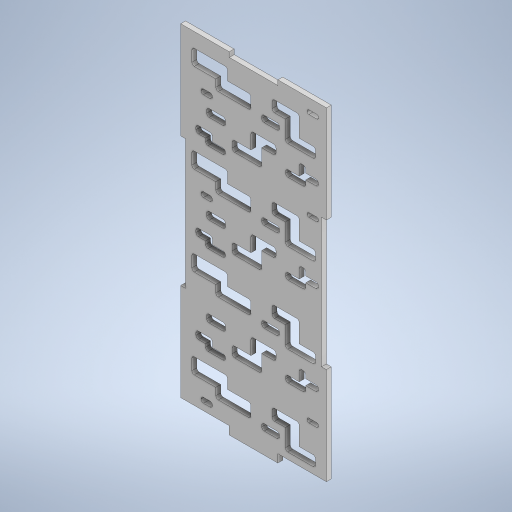
# Autodesk Inventor part: Pièce Ve1
Saved by Autodesk Inventor 2023 (Build 270158000, 158)
## iProperties
Created: 2025-01-14
Part Number: Pièce Ve1
Material: Générique
Document SubType Name: Modeling
Designer: kfadieieva
Density: 1 g/cm^3
Appearance: Par défaut
Author: kfadieieva
Autodesk Inventor part; units mm, degrees
ref_plane "YZ Plane" through (0, 0, 0) normal (1, 0, 0) x (0, 1, 0)
ref_plane "XZ Plane" through (0, 0, 0) normal (0, 1, 0) x (-1, 0, 0)
ref_plane "XY Plane" through (0, 0, 0) normal (0, 0, 1) x (1, 0, 0)
sketch "Esquisse1" plane through (0, 0, 0) normal (0, 0, 1) x (1, 0, 0)
  line L0 (30, 200) -> (30, 197)
  line L1 (30, 197) -> (60, 197)
  line L2 (60, 197) -> (60, 200)
  line L3 (90, 140) -> (87, 140)
  line L4 (87, 140) -> (87, 60)
  line L5 (87, 60) -> (90, 60)
  line L6 (0, 140) -> (3, 140)
  line L7 (3, 140) -> (3, 60)
  line L8 (3, 60) -> (0, 60)
  line L9 (0, 200) -> (0, 140)
  line L10 (0, 60) -> (0, 0)
  line L11 (90, 0) -> (90, 60)
  line L12 (90, 140) -> (90, 200)
  line L13 (90, 200) -> (60, 200)
  line L14 (30, 200) -> (0, 200)
  line L15 (60, 0) -> (60, -5)
  line L16 (60, -5) -> (30, -5)
  line L17 (30, -5) -> (30, 0)
  line L18 (0, 0) -> (30, 0)
  line L19 (60, 0) -> (90, 0)
  dimension "d0" = 90
  dimension "d1" = 200
  dimension "d6" = 200
  dimension "d11" = 3
  dimension "d12" = 3
  dimension "d29" = 30
  dimension "d30" = 3
  dimension "d32" = 30
  dimension "d33" = 30
  dimension "d34" = 90
  dimension "d35" = 90
  dimension "d36" = 90
  dimension "d37" = 90
  dimension "d38" = 90
  dimension "d39" = 90
  dimension "d40" = 90
  dimension "d41" = 5
  dimension "d42" = 90
  dimension "d43" = 90
  dimension "d44" = 90
  dimension "d45" = 90
  dimension "d46" = 90
  constraints: 40 end point, 10 perpendicular, 8 parallel, 3 horizontal, 2 point on line, 1 vertical
  measures "d0" distance of L12.end L9.start
  measures "d1" distance of L11.start L12.end
  measures "d6" distance of L9.start L10.end
  measures "d11" distance of L3.start L3.end
  measures "d12" distance of L1.end L2.end
  measures "d29" distance from line of L9 L0.start
  measures "d30" distance of L6.start L6.end
  measures "d32" distance from line of L16.end L10
  measures "d33" distance from line of L11 L15.end
  measures "d34" angle of L12 L13
  measures "d35" angle of L9 L14
  measures "d36" angle of L0 L14
  measures "d37" angle of L13 L2
  measures "d38" angle of L6 L9
  measures "d39" angle of L10 L8
  measures "d40" angle of L18 L10
  measures "d41" distance of L16.end L17.end
  measures "d42" angle of L19 L15
  measures "d43" angle of L17 L18
  measures "d44" angle of L11 L19
  measures "d45" angle of L11 L5
  measures "d46" angle of L12 L3
extrude "Extrusion1" add sketch "Esquisse1" along normal blind 3
sketch "Esquisse2" plane through (0, 0, 3) normal (0, 0, 1) x (1, 0, 0)
  line L0 (8.393, 191.0718) -> (27.4432, 191.0718)
  line L1 (28.9432, 189.5718) -> (28.9432, 183.8393)
  line L2 (21.7107, 181.3697) -> (8.393, 181.3697)
  line L3 (6.893, 182.8697) -> (6.893, 189.5718)
  line L4 (23.2107, 175.372) -> (41.9082, 175.372)
  line L5 (43.4082, 176.872) -> (43.4082, 182.3393)
  line L6 (41.9082, 183.8393) -> (28.9432, 183.8393)
  line L7 (21.7107, 181.3697) -> (21.7107, 176.872)
  line L8 (57.9619, 188.2494) -> (71.7201, 188.2494)
  line L9 (73.2201, 186.7494) -> (73.2201, 181.3697)
  line L10 (73.2201, 181.3697) -> (57.9619, 181.3697)
  line L11 (56.4619, 182.8697) -> (56.4619, 186.7494)
  line L12 (64.664, 186.2208) -> (73.2201, 186.2208)
  line L13 (73.2201, 186.2208) -> (73.2201, 169.0216)
  line L14 (73.2201, 169.0216) -> (66.164, 169.0216)
  line L15 (64.664, 170.5216) -> (64.664, 186.2208)
  line L16 (69.6921, 169.0216) -> (81.775, 169.0216)
  line L17 (83.275, 170.5216) -> (83.275, 173.872)
  line L18 (81.775, 175.372) -> (69.6921, 175.372)
  line L19 (69.6921, 175.372) -> (69.6921, 169.0216)
  line L20 (14.0378, 172.1968) -> (18.0939, 172.1968)
  line L21 (19.5939, 170.6968) -> (19.5939, 170.5216)
  line L22 (18.0939, 169.0216) -> (14.0378, 169.0216)
  line L23 (12.5378, 170.5216) -> (12.5378, 170.6968)
  line L24 (44.9082, 164.3786) -> (57.362, 164.3786)
  line L25 (58.862, 162.8786) -> (58.862, 160.2175)
  line L26 (57.362, 158.7175) -> (50.0557, 158.7175)
  line L27 (43.4082, 158.7175) -> (43.4082, 162.8786)
  line L28 (50.0557, 158.7175) -> (50.0557, 149.3984)
  line L29 (48.5557, 147.8984) -> (43.4082, 147.8984)
  line L30 (43.4082, 154.1885) -> (43.4082, 162.24)
  line L31 (45.401, 147.8984) -> (33.3142, 147.8984)
  line L32 (31.8142, 149.3984) -> (31.8142, 152.6885)
  line L33 (33.3142, 154.1885) -> (43.4082, 154.1885)
  line L34 (66.341, 155.0692) -> (73.2201, 155.0692)
  line L35 (77.2292, 155.0692) -> (77.2292, 152.5435)
  line L36 (75.7292, 151.0435) -> (66.341, 151.0435)
  line L37 (64.841, 152.5435) -> (64.841, 153.5692)
  line L38 (73.2201, 155.0692) -> (73.2201, 160.798)
  line L39 (74.7201, 162.298) -> (75.7292, 162.298)
  line L40 (77.2292, 158.7175) -> (83.529, 158.7175)
  line L41 (85.029, 157.2175) -> (85.029, 156.5692)
  line L42 (83.529, 155.0692) -> (77.2292, 155.0692)
  line L43 (26.1359, 163.4585) -> (17.5659, 163.4585)
  line L44 (16.0659, 161.9585) -> (16.0659, 160.2175)
  line L45 (17.5659, 158.7175) -> (26.1359, 158.7175)
  line L46 (27.6359, 160.2175) -> (27.6359, 161.9585)
  line L47 (10.9302, 151.0435) -> (18.0939, 151.0435)
  line L48 (19.5939, 149.5435) -> (19.5939, 146.5532)
  line L49 (15.3904, 146.5532) -> (10.9302, 146.5532)
  line L50 (9.4302, 148.0532) -> (9.4302, 149.5435)
  line L51 (19.5939, 146.5532) -> (26.1359, 146.5532)
  line L52 (27.6359, 145.0532) -> (27.6359, 144.6939)
  line L53 (26.1359, 143.1939) -> (16.8904, 143.1939)
  line L54 (15.3904, 144.6939) -> (15.3904, 146.5532)
  line L55 (79.141, 193.6205) -> (84.029, 193.6205)
  line L56 (85.029, 192.6205) -> (85.029, 192.0718)
  line L57 (84.029, 191.0718) -> (79.141, 191.0718)
  line L58 (78.141, 192.0718) -> (78.141, 192.6205)
  arc A0 (8.393, 191.0718) -> (6.893, 189.5718) centre (8.393, 189.5718) ccw
  arc A1 (6.893, 182.8697) -> (8.393, 181.3697) centre (8.393, 182.8697) ccw
  arc A2 (14.0378, 172.1968) -> (12.5378, 170.6968) centre (14.0378, 170.6968) ccw
  arc A3 (12.5378, 170.5216) -> (14.0378, 169.0216) centre (14.0378, 170.5216) ccw
  arc A4 (19.5939, 170.6968) -> (18.0939, 172.1968) centre (18.0939, 170.6968) ccw
  arc A5 (18.0939, 169.0216) -> (19.5939, 170.5216) centre (18.0939, 170.5216) ccw
  arc A6 (27.6359, 161.9585) -> (26.1359, 163.4585) centre (26.1359, 161.9585) ccw
  arc A7 (26.1359, 158.7175) -> (27.6359, 160.2175) centre (26.1359, 160.2175) ccw
  arc A8 (16.0659, 160.2175) -> (17.5659, 158.7175) centre (17.5659, 160.2175) ccw
  arc A9 (17.5659, 163.4585) -> (16.0659, 161.9585) centre (17.5659, 161.9585) ccw
  arc A10 (10.9302, 151.0435) -> (9.4302, 149.5435) centre (10.9302, 149.5435) ccw
  arc A11 (9.4302, 148.0532) -> (10.9302, 146.5532) centre (10.9302, 148.0532) ccw
  arc A12 (19.5939, 149.5435) -> (18.0939, 151.0435) centre (18.0939, 149.5435) ccw
  arc A13 (15.3904, 144.6939) -> (16.8904, 143.1939) centre (16.8904, 144.6939) ccw
  arc A14 (26.1359, 143.1939) -> (27.6359, 144.6939) centre (26.1359, 144.6939) ccw
  arc A15 (27.6359, 145.0532) -> (26.1359, 146.5532) centre (26.1359, 145.0532) ccw
  arc A16 (33.3142, 154.1885) -> (31.8142, 152.6885) centre (33.3142, 152.6885) ccw
  arc A17 (31.8142, 149.3984) -> (33.3142, 147.8984) centre (33.3142, 149.3984) ccw
  arc A18 (44.9082, 164.3786) -> (43.4082, 162.8786) centre (44.9082, 162.8786) ccw
  arc A19 (57.362, 158.7175) -> (58.862, 160.2175) centre (57.362, 160.2175) ccw
  arc A20 (58.862, 162.8786) -> (57.362, 164.3786) centre (57.362, 162.8786) ccw
  arc A21 (48.5557, 147.8984) -> (50.0557, 149.3984) centre (48.5557, 149.3984) ccw
  arc A22 (66.341, 155.0692) -> (64.841, 153.5692) centre (66.341, 153.5692) ccw
  arc A23 (64.841, 152.5435) -> (66.341, 151.0435) centre (66.341, 152.5435) ccw
  arc A24 (75.7292, 151.0435) -> (77.2292, 152.5435) centre (75.7292, 152.5435) ccw
  arc A25 (83.529, 155.0692) -> (85.029, 156.5692) centre (83.529, 156.5692) ccw
  arc A26 (85.029, 157.2175) -> (83.529, 158.7175) centre (83.529, 157.2175) ccw
  arc A27 (77.2292, 160.798) -> (75.7292, 162.298) centre (75.7292, 160.798) ccw
  arc A28 (74.7201, 162.298) -> (73.2201, 160.798) centre (74.7201, 160.798) ccw
  arc A29 (28.9432, 189.5718) -> (27.4432, 191.0718) centre (27.4432, 189.5718) ccw
  arc A30 (21.7107, 176.872) -> (23.2107, 175.372) centre (23.2107, 176.872) ccw
  arc A31 (41.9082, 175.372) -> (43.4082, 176.872) centre (41.9082, 176.872) ccw
  arc A32 (43.4082, 182.3393) -> (41.9082, 183.8393) centre (41.9082, 182.3393) ccw
  arc A33 (57.9619, 188.2494) -> (56.4619, 186.7494) centre (57.9619, 186.7494) ccw
  arc A34 (56.4619, 182.8697) -> (57.9619, 181.3697) centre (57.9619, 182.8697) ccw
  arc A35 (73.2201, 186.7494) -> (71.7201, 188.2494) centre (71.7201, 186.7494) ccw
  arc A36 (64.664, 170.5216) -> (66.164, 169.0216) centre (66.164, 170.5216) ccw
  arc A37 (81.775, 169.0216) -> (83.275, 170.5216) centre (81.775, 170.5216) ccw
  arc A38 (83.275, 173.872) -> (81.775, 175.372) centre (81.775, 173.872) ccw
  line L59 (51.5557, 176.872) -> (59.471, 176.872)
  line L60 (60.971, 175.372) -> (60.971, 174.415)
  line L61 (59.471, 172.915) -> (51.5557, 172.915)
  line L62 (50.0557, 174.415) -> (50.0557, 175.372)
  arc A39 (51.5557, 176.872) -> (50.0557, 175.372) centre (51.5557, 175.372) ccw
  arc A40 (50.0557, 174.415) -> (51.5557, 172.915) centre (51.5557, 174.415) ccw
  arc A41 (59.471, 172.915) -> (60.971, 174.415) centre (59.471, 174.415) ccw
  arc A42 (60.971, 175.372) -> (59.471, 176.872) centre (59.471, 175.372) ccw
  arc A43 (79.141, 193.6205) -> (78.141, 192.6205) centre (79.141, 192.6205) ccw
  arc A44 (78.141, 192.0718) -> (79.141, 191.0718) centre (79.141, 192.0718) ccw
  arc A45 (85.029, 192.6205) -> (84.029, 193.6205) centre (84.029, 192.6205) ccw
  arc A46 (84.029, 191.0718) -> (85.029, 192.0718) centre (84.029, 192.0718) ccw
  line L63 (43.4082, 162.24) -> (43.5509, 162.24)
  line L64 (77.2292, 160.798) -> (77.2292, 158.7175)
  line L65 (77.2292, 155.0692) -> (77.2292, 153.8063)
  arc A47 (6.893, 127.8697) -> (8.393, 126.3697) centre (8.393, 127.8697) ccw
  line L66 (6.893, 127.8697) -> (6.893, 134.5718)
  arc A48 (8.393, 136.0718) -> (6.893, 134.5718) centre (8.393, 134.5718) ccw
  line L67 (12.5378, 115.5216) -> (12.5378, 115.6968)
  line L68 (66.341, 100.0692) -> (73.2201, 100.0692)
  line L69 (77.2292, 100.0692) -> (77.2292, 97.5435)
  line L70 (75.7292, 96.0435) -> (66.341, 96.0435)
  line L71 (77.2292, 100.0692) -> (77.2292, 98.8063)
  arc A49 (75.7292, 96.0435) -> (77.2292, 97.5435) centre (75.7292, 97.5435) ccw
  line L72 (83.529, 100.0692) -> (77.2292, 100.0692)
  line L73 (77.2292, 105.798) -> (77.2292, 103.7175)
  line L74 (73.2201, 100.0692) -> (73.2201, 105.798)
  line L75 (74.7201, 107.298) -> (75.7292, 107.298)
  arc A50 (74.7201, 107.298) -> (73.2201, 105.798) centre (74.7201, 105.798) ccw
  arc A51 (77.2292, 105.798) -> (75.7292, 107.298) centre (75.7292, 105.798) ccw
  line L76 (77.2292, 103.7175) -> (83.529, 103.7175)
  line L77 (10.9302, 96.0435) -> (18.0939, 96.0435)
  line L78 (15.3904, 91.5532) -> (10.9302, 91.5532)
  line L79 (9.4302, 93.0532) -> (9.4302, 94.5435)
  arc A52 (10.9302, 96.0435) -> (9.4302, 94.5435) centre (10.9302, 94.5435) ccw
  arc A53 (9.4302, 93.0532) -> (10.9302, 91.5532) centre (10.9302, 93.0532) ccw
  line L80 (15.3904, 89.6939) -> (15.3904, 91.5532)
  line L81 (57.9619, 133.2494) -> (71.7201, 133.2494)
  line L82 (73.2201, 131.7494) -> (73.2201, 126.3697)
  line L83 (73.2201, 126.3697) -> (57.9619, 126.3697)
  line L84 (64.664, 131.2208) -> (73.2201, 131.2208)
  line L85 (73.2201, 131.2208) -> (73.2201, 114.0216)
  line L86 (73.2201, 114.0216) -> (66.164, 114.0216)
  line L87 (64.664, 115.5216) -> (64.664, 131.2208)
  line L88 (69.6921, 114.0216) -> (81.775, 114.0216)
  line L89 (83.275, 115.5216) -> (83.275, 118.872)
  line L90 (81.775, 120.372) -> (69.6921, 120.372)
  line L91 (69.6921, 120.372) -> (69.6921, 114.0216)
  arc A54 (73.2201, 131.7494) -> (71.7201, 133.2494) centre (71.7201, 131.7494) ccw
  arc A55 (83.275, 118.872) -> (81.775, 120.372) centre (81.775, 118.872) ccw
  arc A56 (81.775, 114.0216) -> (83.275, 115.5216) centre (81.775, 115.5216) ccw
  arc A57 (14.0378, 117.1968) -> (12.5378, 115.6968) centre (14.0378, 115.6968) ccw
  arc A58 (12.5378, 115.5216) -> (14.0378, 114.0216) centre (14.0378, 115.5216) ccw
  line L92 (8.393, 136.0718) -> (27.4432, 136.0718)
  line L93 (21.7107, 126.3697) -> (8.393, 126.3697)
  line L94 (14.0378, 117.1968) -> (18.0939, 117.1968)
  arc A59 (19.5939, 115.6968) -> (18.0939, 117.1968) centre (18.0939, 115.6968) ccw
  line L95 (19.5939, 115.6968) -> (19.5939, 115.5216)
  line L96 (18.0939, 114.0216) -> (14.0378, 114.0216)
  arc A60 (18.0939, 114.0216) -> (19.5939, 115.5216) centre (18.0939, 115.5216) ccw
  line L97 (26.1359, 108.4585) -> (17.5659, 108.4585)
  line L98 (16.0659, 106.9585) -> (16.0659, 105.2175)
  line L99 (17.5659, 103.7175) -> (26.1359, 103.7175)
  line L100 (27.6359, 105.2175) -> (27.6359, 106.9585)
  arc A61 (17.5659, 108.4585) -> (16.0659, 106.9585) centre (17.5659, 106.9585) ccw
  arc A62 (16.0659, 105.2175) -> (17.5659, 103.7175) centre (17.5659, 105.2175) ccw
  arc A63 (27.6359, 106.9585) -> (26.1359, 108.4585) centre (26.1359, 106.9585) ccw
  arc A64 (26.1359, 103.7175) -> (27.6359, 105.2175) centre (26.1359, 105.2175) ccw
  line L101 (44.9082, 109.3786) -> (57.362, 109.3786)
  line L102 (58.862, 107.8786) -> (58.862, 105.2175)
  line L103 (57.362, 103.7175) -> (50.0557, 103.7175)
  line L104 (64.841, 97.5435) -> (64.841, 98.5692)
  arc A65 (57.362, 103.7175) -> (58.862, 105.2175) centre (57.362, 105.2175) ccw
  arc A66 (58.862, 107.8786) -> (57.362, 109.3786) centre (57.362, 107.8786) ccw
  arc A67 (66.341, 100.0692) -> (64.841, 98.5692) centre (66.341, 98.5692) ccw
  arc A68 (64.664, 115.5216) -> (66.164, 114.0216) centre (66.164, 115.5216) ccw
  arc A69 (64.841, 97.5435) -> (66.341, 96.0435) centre (66.341, 97.5435) ccw
  line L105 (28.9432, 134.5718) -> (28.9432, 128.8393)
  line L106 (23.2107, 120.372) -> (41.9082, 120.372)
  line L107 (43.4082, 121.872) -> (43.4082, 127.3393)
  line L108 (41.9082, 128.8393) -> (28.9432, 128.8393)
  line L109 (21.7107, 126.3697) -> (21.7107, 121.872)
  arc A70 (28.9432, 134.5718) -> (27.4432, 136.0718) centre (27.4432, 134.5718) ccw
  arc A71 (21.7107, 121.872) -> (23.2107, 120.372) centre (23.2107, 121.872) ccw
  arc A72 (41.9082, 120.372) -> (43.4082, 121.872) centre (41.9082, 121.872) ccw
  arc A73 (43.4082, 127.3393) -> (41.9082, 128.8393) centre (41.9082, 127.3393) ccw
  line L110 (56.4619, 127.8697) -> (56.4619, 131.7494)
  line L111 (50.0557, 119.415) -> (50.0557, 120.372)
  arc A74 (51.5557, 121.872) -> (50.0557, 120.372) centre (51.5557, 120.372) ccw
  arc A75 (50.0557, 119.415) -> (51.5557, 117.915) centre (51.5557, 119.415) ccw
  arc A76 (57.9619, 133.2494) -> (56.4619, 131.7494) centre (57.9619, 131.7494) ccw
  arc A77 (56.4619, 127.8697) -> (57.9619, 126.3697) centre (57.9619, 127.8697) ccw
  line L112 (51.5557, 121.872) -> (59.471, 121.872)
  line L113 (59.471, 117.915) -> (51.5557, 117.915)
  line L114 (60.971, 120.372) -> (60.971, 119.415)
  arc A78 (59.471, 117.915) -> (60.971, 119.415) centre (59.471, 119.415) ccw
  arc A79 (60.971, 120.372) -> (59.471, 121.872) centre (59.471, 120.372) ccw
  line L115 (43.4082, 103.7175) -> (43.4082, 107.8786)
  line L116 (50.0557, 103.7175) -> (50.0557, 94.3984)
  line L117 (48.5557, 92.8984) -> (43.4082, 92.8984)
  line L118 (43.4082, 99.1885) -> (43.4082, 107.24)
  line L119 (45.401, 92.8984) -> (33.3142, 92.8984)
  line L120 (31.8142, 94.3984) -> (31.8142, 97.6885)
  line L121 (33.3142, 99.1885) -> (43.4082, 99.1885)
  arc A80 (33.3142, 99.1885) -> (31.8142, 97.6885) centre (33.3142, 97.6885) ccw
  arc A81 (31.8142, 94.3984) -> (33.3142, 92.8984) centre (33.3142, 94.3984) ccw
  arc A82 (44.9082, 109.3786) -> (43.4082, 107.8786) centre (44.9082, 107.8786) ccw
  arc A83 (48.5557, 92.8984) -> (50.0557, 94.3984) centre (48.5557, 94.3984) ccw
  line L122 (43.4082, 107.24) -> (43.5509, 107.24)
  line L123 (19.5939, 94.5435) -> (19.5939, 91.5532)
  arc A84 (15.3904, 89.6939) -> (16.8904, 88.1939) centre (16.8904, 89.6939) ccw
  arc A85 (19.5939, 94.5435) -> (18.0939, 96.0435) centre (18.0939, 94.5435) ccw
  line L124 (26.1359, 88.1939) -> (16.8904, 88.1939)
  line L125 (19.5939, 91.5532) -> (26.1359, 91.5532)
  arc A86 (27.6359, 90.0532) -> (26.1359, 91.5532) centre (26.1359, 90.0532) ccw
  line L126 (27.6359, 90.0532) -> (27.6359, 89.6939)
  arc A87 (26.1359, 88.1939) -> (27.6359, 89.6939) centre (26.1359, 89.6939) ccw
  arc A88 (85.029, 102.2175) -> (83.529, 103.7175) centre (83.529, 102.2175) ccw
  line L127 (85.029, 102.2175) -> (85.029, 101.5692)
  arc A89 (83.529, 100.0692) -> (85.029, 101.5692) centre (83.529, 101.5692) ccw
  line L128 (84.029, 136.0718) -> (79.141, 136.0718)
  arc A90 (78.141, 137.0718) -> (79.141, 136.0718) centre (79.141, 137.0718) ccw
  line L129 (78.141, 137.0718) -> (78.141, 137.6205)
  arc A91 (84.029, 136.0718) -> (85.029, 137.0718) centre (84.029, 137.0718) ccw
  line L130 (85.029, 137.6205) -> (85.029, 137.0718)
  line L131 (79.141, 138.6205) -> (84.029, 138.6205)
  arc A92 (85.029, 137.6205) -> (84.029, 138.6205) centre (84.029, 137.6205) ccw
  arc A93 (79.141, 138.6205) -> (78.141, 137.6205) centre (79.141, 137.6205) ccw
  arc A94 (6.893, 72.8697) -> (8.393, 71.3697) centre (8.393, 72.8697) ccw
  line L132 (6.893, 72.8697) -> (6.893, 79.5718)
  arc A95 (8.393, 81.0718) -> (6.893, 79.5718) centre (8.393, 79.5718) ccw
  line L133 (12.5378, 60.5216) -> (12.5378, 60.6968)
  line L134 (66.341, 45.0692) -> (73.2201, 45.0692)
  line L135 (77.2292, 45.0692) -> (77.2292, 42.5435)
  line L136 (75.7292, 41.0435) -> (66.341, 41.0435)
  line L137 (77.2292, 45.0692) -> (77.2292, 43.8063)
  arc A96 (75.7292, 41.0435) -> (77.2292, 42.5435) centre (75.7292, 42.5435) ccw
  line L138 (83.529, 45.0692) -> (77.2292, 45.0692)
  line L139 (77.2292, 50.798) -> (77.2292, 48.7175)
  line L140 (73.2201, 45.0692) -> (73.2201, 50.798)
  line L141 (74.7201, 52.298) -> (75.7292, 52.298)
  arc A97 (74.7201, 52.298) -> (73.2201, 50.798) centre (74.7201, 50.798) ccw
  arc A98 (77.2292, 50.798) -> (75.7292, 52.298) centre (75.7292, 50.798) ccw
  line L142 (77.2292, 48.7175) -> (83.529, 48.7175)
  line L143 (10.9302, 41.0435) -> (18.0939, 41.0435)
  line L144 (15.3904, 36.5532) -> (10.9302, 36.5532)
  line L145 (9.4302, 38.0532) -> (9.4302, 39.5435)
  arc A99 (10.9302, 41.0435) -> (9.4302, 39.5435) centre (10.9302, 39.5435) ccw
  arc A100 (9.4302, 38.0532) -> (10.9302, 36.5532) centre (10.9302, 38.0532) ccw
  line L146 (15.3904, 34.6939) -> (15.3904, 36.5532)
  line L147 (57.9619, 78.2494) -> (71.7201, 78.2494)
  line L148 (73.2201, 76.7494) -> (73.2201, 71.3697)
  line L149 (73.2201, 71.3697) -> (57.9619, 71.3697)
  line L150 (64.664, 76.2208) -> (73.2201, 76.2208)
  line L151 (73.2201, 76.2208) -> (73.2201, 59.0216)
  line L152 (73.2201, 59.0216) -> (66.164, 59.0216)
  line L153 (64.664, 60.5216) -> (64.664, 76.2208)
  line L154 (69.6921, 59.0216) -> (81.775, 59.0216)
  line L155 (83.275, 60.5216) -> (83.275, 63.872)
  line L156 (81.775, 65.372) -> (69.6921, 65.372)
  line L157 (69.6921, 65.372) -> (69.6921, 59.0216)
  arc A101 (73.2201, 76.7494) -> (71.7201, 78.2494) centre (71.7201, 76.7494) ccw
  arc A102 (83.275, 63.872) -> (81.775, 65.372) centre (81.775, 63.872) ccw
  arc A103 (81.775, 59.0216) -> (83.275, 60.5216) centre (81.775, 60.5216) ccw
  arc A104 (14.0378, 62.1968) -> (12.5378, 60.6968) centre (14.0378, 60.6968) ccw
  arc A105 (12.5378, 60.5216) -> (14.0378, 59.0216) centre (14.0378, 60.5216) ccw
  line L158 (8.393, 81.0718) -> (27.4432, 81.0718)
  line L159 (21.7107, 71.3697) -> (8.393, 71.3697)
  line L160 (14.0378, 62.1968) -> (18.0939, 62.1968)
  arc A106 (19.5939, 60.6968) -> (18.0939, 62.1968) centre (18.0939, 60.6968) ccw
  line L161 (19.5939, 60.6968) -> (19.5939, 60.5216)
  line L162 (18.0939, 59.0216) -> (14.0378, 59.0216)
  arc A107 (18.0939, 59.0216) -> (19.5939, 60.5216) centre (18.0939, 60.5216) ccw
  line L163 (26.1359, 53.4585) -> (17.5659, 53.4585)
  line L164 (16.0659, 51.9585) -> (16.0659, 50.2175)
  line L165 (17.5659, 48.7175) -> (26.1359, 48.7175)
  line L166 (27.6359, 50.2175) -> (27.6359, 51.9585)
  arc A108 (17.5659, 53.4585) -> (16.0659, 51.9585) centre (17.5659, 51.9585) ccw
  arc A109 (16.0659, 50.2175) -> (17.5659, 48.7175) centre (17.5659, 50.2175) ccw
  arc A110 (27.6359, 51.9585) -> (26.1359, 53.4585) centre (26.1359, 51.9585) ccw
  arc A111 (26.1359, 48.7175) -> (27.6359, 50.2175) centre (26.1359, 50.2175) ccw
  line L167 (44.9082, 54.3786) -> (57.362, 54.3786)
  line L168 (58.862, 52.8786) -> (58.862, 50.2175)
  line L169 (57.362, 48.7175) -> (50.0557, 48.7175)
  line L170 (64.841, 42.5435) -> (64.841, 43.5692)
  arc A112 (57.362, 48.7175) -> (58.862, 50.2175) centre (57.362, 50.2175) ccw
  arc A113 (58.862, 52.8786) -> (57.362, 54.3786) centre (57.362, 52.8786) ccw
  arc A114 (66.341, 45.0692) -> (64.841, 43.5692) centre (66.341, 43.5692) ccw
  arc A115 (64.664, 60.5216) -> (66.164, 59.0216) centre (66.164, 60.5216) ccw
  arc A116 (64.841, 42.5435) -> (66.341, 41.0435) centre (66.341, 42.5435) ccw
  line L171 (28.9432, 79.5718) -> (28.9432, 73.8393)
  line L172 (23.2107, 65.372) -> (41.9082, 65.372)
  line L173 (43.4082, 66.872) -> (43.4082, 72.3393)
  line L174 (41.9082, 73.8393) -> (28.9432, 73.8393)
  line L175 (21.7107, 71.3697) -> (21.7107, 66.872)
  arc A117 (28.9432, 79.5718) -> (27.4432, 81.0718) centre (27.4432, 79.5718) ccw
  arc A118 (21.7107, 66.872) -> (23.2107, 65.372) centre (23.2107, 66.872) ccw
  arc A119 (41.9082, 65.372) -> (43.4082, 66.872) centre (41.9082, 66.872) ccw
  arc A120 (43.4082, 72.3393) -> (41.9082, 73.8393) centre (41.9082, 72.3393) ccw
  line L176 (56.4619, 72.8697) -> (56.4619, 76.7494)
  line L177 (50.0557, 64.415) -> (50.0557, 65.372)
  arc A121 (51.5557, 66.872) -> (50.0557, 65.372) centre (51.5557, 65.372) ccw
  arc A122 (50.0557, 64.415) -> (51.5557, 62.915) centre (51.5557, 64.415) ccw
  arc A123 (57.9619, 78.2494) -> (56.4619, 76.7494) centre (57.9619, 76.7494) ccw
  arc A124 (56.4619, 72.8697) -> (57.9619, 71.3697) centre (57.9619, 72.8697) ccw
  line L178 (51.5557, 66.872) -> (59.471, 66.872)
  line L179 (59.471, 62.915) -> (51.5557, 62.915)
  line L180 (60.971, 65.372) -> (60.971, 64.415)
  arc A125 (59.471, 62.915) -> (60.971, 64.415) centre (59.471, 64.415) ccw
  arc A126 (60.971, 65.372) -> (59.471, 66.872) centre (59.471, 65.372) ccw
  line L181 (43.4082, 48.7175) -> (43.4082, 52.8786)
  line L182 (50.0557, 48.7175) -> (50.0557, 39.3984)
  line L183 (48.5557, 37.8984) -> (43.4082, 37.8984)
  line L184 (43.4082, 44.1885) -> (43.4082, 52.24)
  line L185 (45.401, 37.8984) -> (33.3142, 37.8984)
  line L186 (31.8142, 39.3984) -> (31.8142, 42.6885)
  line L187 (33.3142, 44.1885) -> (43.4082, 44.1885)
  arc A127 (33.3142, 44.1885) -> (31.8142, 42.6885) centre (33.3142, 42.6885) ccw
  arc A128 (31.8142, 39.3984) -> (33.3142, 37.8984) centre (33.3142, 39.3984) ccw
  arc A129 (44.9082, 54.3786) -> (43.4082, 52.8786) centre (44.9082, 52.8786) ccw
  arc A130 (48.5557, 37.8984) -> (50.0557, 39.3984) centre (48.5557, 39.3984) ccw
  line L188 (43.4082, 52.24) -> (43.5509, 52.24)
  line L189 (19.5939, 39.5435) -> (19.5939, 36.5532)
  arc A131 (15.3904, 34.6939) -> (16.8904, 33.1939) centre (16.8904, 34.6939) ccw
  arc A132 (19.5939, 39.5435) -> (18.0939, 41.0435) centre (18.0939, 39.5435) ccw
  line L190 (26.1359, 33.1939) -> (16.8904, 33.1939)
  line L191 (19.5939, 36.5532) -> (26.1359, 36.5532)
  arc A133 (27.6359, 35.0532) -> (26.1359, 36.5532) centre (26.1359, 35.0532) ccw
  line L192 (27.6359, 35.0532) -> (27.6359, 34.6939)
  arc A134 (26.1359, 33.1939) -> (27.6359, 34.6939) centre (26.1359, 34.6939) ccw
  arc A135 (85.029, 47.2175) -> (83.529, 48.7175) centre (83.529, 47.2175) ccw
  line L193 (85.029, 47.2175) -> (85.029, 46.5692)
  arc A136 (83.529, 45.0692) -> (85.029, 46.5692) centre (83.529, 46.5692) ccw
  line L194 (84.029, 81.0718) -> (79.141, 81.0718)
  arc A137 (78.141, 82.0718) -> (79.141, 81.0718) centre (79.141, 82.0718) ccw
  line L195 (78.141, 82.0718) -> (78.141, 82.6205)
  arc A138 (84.029, 81.0718) -> (85.029, 82.0718) centre (84.029, 82.0718) ccw
  line L196 (85.029, 82.6205) -> (85.029, 82.0718)
  line L197 (79.141, 83.6205) -> (84.029, 83.6205)
  arc A139 (85.029, 82.6205) -> (84.029, 83.6205) centre (84.029, 82.6205) ccw
  arc A140 (79.141, 83.6205) -> (78.141, 82.6205) centre (79.141, 82.6205) ccw
  arc A141 (6.893, 17.8697) -> (8.393, 16.3697) centre (8.393, 17.8697) ccw
  line L198 (6.893, 17.8697) -> (6.893, 24.5718)
  arc A142 (8.393, 26.0718) -> (6.893, 24.5718) centre (8.393, 24.5718) ccw
  line L199 (12.5378, 5.5216) -> (12.5378, 5.6968)
  line L200 (66.341, -9.9308) -> (73.2201, -9.9308)
  line L201 (77.2292, -9.9308) -> (77.2292, -12.4565)
  line L202 (75.7292, -13.9565) -> (66.341, -13.9565)
  line L203 (77.2292, -9.9308) -> (77.2292, -11.1937)
  arc A143 (75.7292, -13.9565) -> (77.2292, -12.4565) centre (75.7292, -12.4565) ccw
  line L204 (83.529, -9.9308) -> (77.2292, -9.9308)
  line L205 (77.2292, -4.202) -> (77.2292, -6.2825)
  line L206 (73.2201, -9.9308) -> (73.2201, -4.202)
  line L207 (74.7201, -2.702) -> (75.7292, -2.702)
  arc A144 (74.7201, -2.702) -> (73.2201, -4.202) centre (74.7201, -4.202) ccw
  arc A145 (77.2292, -4.202) -> (75.7292, -2.702) centre (75.7292, -4.202) ccw
  line L208 (77.2292, -6.2825) -> (83.529, -6.2825)
  line L209 (10.9302, -13.9565) -> (18.0939, -13.9565)
  line L210 (15.3904, -18.4468) -> (10.9302, -18.4468)
  line L211 (9.4302, -16.9468) -> (9.4302, -15.4565)
  arc A146 (10.9302, -13.9565) -> (9.4302, -15.4565) centre (10.9302, -15.4565) ccw
  arc A147 (9.4302, -16.9468) -> (10.9302, -18.4468) centre (10.9302, -16.9468) ccw
  line L212 (15.3904, -20.3061) -> (15.3904, -18.4468)
  line L213 (57.9619, 23.2494) -> (71.7201, 23.2494)
  line L214 (73.2201, 21.7494) -> (73.2201, 16.3697)
  line L215 (73.2201, 16.3697) -> (57.9619, 16.3697)
  line L216 (64.664, 21.2208) -> (73.2201, 21.2208)
  line L217 (73.2201, 21.2208) -> (73.2201, 4.0216)
  line L218 (73.2201, 4.0216) -> (66.164, 4.0216)
  line L219 (64.664, 5.5216) -> (64.664, 21.2208)
  line L220 (69.6921, 4.0216) -> (81.775, 4.0216)
  line L221 (83.275, 5.5216) -> (83.275, 8.872)
  line L222 (81.775, 10.372) -> (69.6921, 10.372)
  line L223 (69.6921, 10.372) -> (69.6921, 4.0216)
  arc A148 (73.2201, 21.7494) -> (71.7201, 23.2494) centre (71.7201, 21.7494) ccw
  arc A149 (83.275, 8.872) -> (81.775, 10.372) centre (81.775, 8.872) ccw
  arc A150 (81.775, 4.0216) -> (83.275, 5.5216) centre (81.775, 5.5216) ccw
  arc A151 (14.0378, 7.1968) -> (12.5378, 5.6968) centre (14.0378, 5.6968) ccw
  arc A152 (12.5378, 5.5216) -> (14.0378, 4.0216) centre (14.0378, 5.5216) ccw
  line L224 (8.393, 26.0718) -> (27.4432, 26.0718)
  line L225 (21.7107, 16.3697) -> (8.393, 16.3697)
  line L226 (14.0378, 7.1968) -> (18.0939, 7.1968)
  arc A153 (19.5939, 5.6968) -> (18.0939, 7.1968) centre (18.0939, 5.6968) ccw
  line L227 (19.5939, 5.6968) -> (19.5939, 5.5216)
  line L228 (18.0939, 4.0216) -> (14.0378, 4.0216)
  arc A154 (18.0939, 4.0216) -> (19.5939, 5.5216) centre (18.0939, 5.5216) ccw
  line L229 (26.1359, -1.5415) -> (17.5659, -1.5415)
  line L230 (16.0659, -3.0415) -> (16.0659, -4.7825)
  line L231 (17.5659, -6.2825) -> (26.1359, -6.2825)
  line L232 (27.6359, -4.7825) -> (27.6359, -3.0415)
  arc A155 (17.5659, -1.5415) -> (16.0659, -3.0415) centre (17.5659, -3.0415) ccw
  arc A156 (16.0659, -4.7825) -> (17.5659, -6.2825) centre (17.5659, -4.7825) ccw
  arc A157 (27.6359, -3.0415) -> (26.1359, -1.5415) centre (26.1359, -3.0415) ccw
  arc A158 (26.1359, -6.2825) -> (27.6359, -4.7825) centre (26.1359, -4.7825) ccw
  line L233 (44.9082, -0.6214) -> (57.362, -0.6214)
  line L234 (58.862, -2.1214) -> (58.862, -4.7825)
  line L235 (57.362, -6.2825) -> (50.0557, -6.2825)
  line L236 (64.841, -12.4565) -> (64.841, -11.4308)
  arc A159 (57.362, -6.2825) -> (58.862, -4.7825) centre (57.362, -4.7825) ccw
  arc A160 (58.862, -2.1214) -> (57.362, -0.6214) centre (57.362, -2.1214) ccw
  arc A161 (66.341, -9.9308) -> (64.841, -11.4308) centre (66.341, -11.4308) ccw
  arc A162 (64.664, 5.5216) -> (66.164, 4.0216) centre (66.164, 5.5216) ccw
  arc A163 (64.841, -12.4565) -> (66.341, -13.9565) centre (66.341, -12.4565) ccw
  line L237 (28.9432, 24.5718) -> (28.9432, 18.8393)
  line L238 (23.2107, 10.372) -> (41.9082, 10.372)
  line L239 (43.4082, 11.872) -> (43.4082, 17.3393)
  line L240 (41.9082, 18.8393) -> (28.9432, 18.8393)
  line L241 (21.7107, 16.3697) -> (21.7107, 11.872)
  arc A164 (28.9432, 24.5718) -> (27.4432, 26.0718) centre (27.4432, 24.5718) ccw
  arc A165 (21.7107, 11.872) -> (23.2107, 10.372) centre (23.2107, 11.872) ccw
  arc A166 (41.9082, 10.372) -> (43.4082, 11.872) centre (41.9082, 11.872) ccw
  arc A167 (43.4082, 17.3393) -> (41.9082, 18.8393) centre (41.9082, 17.3393) ccw
  line L242 (56.4619, 17.8697) -> (56.4619, 21.7494)
  line L243 (50.0557, 9.415) -> (50.0557, 10.372)
  arc A168 (51.5557, 11.872) -> (50.0557, 10.372) centre (51.5557, 10.372) ccw
  arc A169 (50.0557, 9.415) -> (51.5557, 7.915) centre (51.5557, 9.415) ccw
  arc A170 (57.9619, 23.2494) -> (56.4619, 21.7494) centre (57.9619, 21.7494) ccw
  arc A171 (56.4619, 17.8697) -> (57.9619, 16.3697) centre (57.9619, 17.8697) ccw
  line L244 (51.5557, 11.872) -> (59.471, 11.872)
  line L245 (59.471, 7.915) -> (51.5557, 7.915)
  line L246 (60.971, 10.372) -> (60.971, 9.415)
  arc A172 (59.471, 7.915) -> (60.971, 9.415) centre (59.471, 9.415) ccw
  arc A173 (60.971, 10.372) -> (59.471, 11.872) centre (59.471, 10.372) ccw
  line L247 (43.4082, -6.2825) -> (43.4082, -2.1214)
  line L248 (50.0557, -6.2825) -> (50.0557, -15.6016)
  line L249 (48.5557, -17.1016) -> (43.4082, -17.1016)
  line L250 (43.4082, -10.8115) -> (43.4082, -2.76)
  line L251 (45.401, -17.1016) -> (33.3142, -17.1016)
  line L252 (31.8142, -15.6016) -> (31.8142, -12.3115)
  line L253 (33.3142, -10.8115) -> (43.4082, -10.8115)
  arc A174 (33.3142, -10.8115) -> (31.8142, -12.3115) centre (33.3142, -12.3115) ccw
  arc A175 (31.8142, -15.6016) -> (33.3142, -17.1016) centre (33.3142, -15.6016) ccw
  arc A176 (44.9082, -0.6214) -> (43.4082, -2.1214) centre (44.9082, -2.1214) ccw
  arc A177 (48.5557, -17.1016) -> (50.0557, -15.6016) centre (48.5557, -15.6016) ccw
  line L254 (43.4082, -2.76) -> (43.5509, -2.76)
  line L255 (19.5939, -15.4565) -> (19.5939, -18.4468)
  arc A178 (15.3904, -20.3061) -> (16.8904, -21.8061) centre (16.8904, -20.3061) ccw
  arc A179 (19.5939, -15.4565) -> (18.0939, -13.9565) centre (18.0939, -15.4565) ccw
  line L256 (26.1359, -21.8061) -> (16.8904, -21.8061)
  line L257 (19.5939, -18.4468) -> (26.1359, -18.4468)
  arc A180 (27.6359, -19.9468) -> (26.1359, -18.4468) centre (26.1359, -19.9468) ccw
  line L258 (27.6359, -19.9468) -> (27.6359, -20.3061)
  arc A181 (26.1359, -21.8061) -> (27.6359, -20.3061) centre (26.1359, -20.3061) ccw
  arc A182 (85.029, -7.7825) -> (83.529, -6.2825) centre (83.529, -7.7825) ccw
  line L259 (85.029, -7.7825) -> (85.029, -8.4308)
  arc A183 (83.529, -9.9308) -> (85.029, -8.4308) centre (83.529, -8.4308) ccw
  line L260 (84.029, 26.0718) -> (79.141, 26.0718)
  arc A184 (78.141, 27.0718) -> (79.141, 26.0718) centre (79.141, 27.0718) ccw
  line L261 (78.141, 27.0718) -> (78.141, 27.6205)
  arc A185 (84.029, 26.0718) -> (85.029, 27.0718) centre (84.029, 27.0718) ccw
  line L262 (85.029, 27.6205) -> (85.029, 27.0718)
  line L263 (79.141, 28.6205) -> (84.029, 28.6205)
  arc A186 (85.029, 27.6205) -> (84.029, 28.6205) centre (84.029, 27.6205) ccw
  arc A187 (79.141, 28.6205) -> (78.141, 27.6205) centre (79.141, 27.6205) ccw
  point P0 (0, 0)
  point P1 (83.275, 175.372)
  point P2 (19.5939, 169.0216)
  point P3 (43.4082, 164.3786)
  point P4 (73.2201, 162.298)
  point P5 (85.029, 155.0692)
  point P6 (16.0659, 158.7175)
  point P7 (9.4302, 151.0435)
  point P8 (27.6359, 143.1939)
  point P9 (85.029, 191.0718)
  point P10 (53.5332, 175.372)
  point P11 (85.029, 100.0692)
  point P12 (9.4302, 96.0435)
  point P13 (73.2201, 107.298)
  point P14 (16.0659, 103.7175)
  point P15 (83.275, 120.372)
  point P16 (19.5939, 114.0216)
  point P17 (53.5332, 120.372)
  point P18 (85.029, 136.0718)
  point P19 (27.6359, 88.1939)
  point P20 (43.4082, 109.3786)
  point P21 (85.029, 45.0692)
  point P22 (9.4302, 41.0435)
  point P23 (73.2201, 52.298)
  point P24 (16.0659, 48.7175)
  point P25 (83.275, 65.372)
  point P26 (19.5939, 59.0216)
  point P27 (53.5332, 65.372)
  point P28 (85.029, 81.0718)
  point P29 (27.6359, 33.1939)
  point P30 (43.4082, 54.3786)
  point P31 (85.029, -9.9308)
  point P32 (9.4302, -13.9565)
  point P33 (73.2201, -2.702)
  point P34 (16.0659, -6.2825)
  point P35 (83.275, 10.372)
  point P36 (19.5939, 4.0216)
  point P37 (53.5332, 10.372)
  point P38 (85.029, 26.0718)
  point P39 (27.6359, -21.8061)
  point P40 (43.4082, -0.6214)
  point P41 (73.2201, 65.372)
  point P42 (64.664, 71.3697)
  point P43 (73.2201, 120.372)
  point P44 (64.664, 126.3697)
  point P45 (73.2201, 175.372)
  point P46 (64.664, 181.3697)
  point P47 (73.2201, 10.372)
  point P48 (64.664, 16.3697)
  dimension "d15" = 1.5
  dimension "d16" = 1.5
  dimension "d17" = 1.5
  dimension "d18" = 1.5
  dimension "d19" = 1
  dimension "d22" = 55
  constraints: 528 end point, 380 point on circle, 188 centre point, 140 point on line, 95 tangent, 42 equal radius, 32 parallel, 16 horizontal, 16 perpendicular, 2 midpoint, 1 collinear, 1 vertical, 854 other
  measures "d15" radius of A0
  measures "d16" radius of A29
  measures "d17" radius of A34
  measures "d18" radius of A39
  measures "d19" radius of A43
  measures "d22" distance of L2.end L93.end
extrude "Extrusion2" cut sketch "Esquisse2" against normal blind 3 contours L0 A29 L1 L6 A32 L5 A31 L4 A30 L7 L2 A1 L3 A0 | L8 A35 L9 L12 L15 L10 A34 L11 A33 | L9 L10 L15 L12 | L13 L18 L19 L14 A36 L15 L10 | L18 A38 L17 A37 L16 L13 | L13 L14 L19 L18 | L20 A4 L21 A5 L22 A3 L23 A2 | L24 A20 L25 A19 L26 L28 A21 L29 L31 A17 L32 A16 L33 L30 L27 A18 | L34 L38 A28 L39 A27 L64 L40 A26 L41 A25 L42 L35 A24 L36 A23 L37 A22 | A6 L46 A7 L45 A8 L44 A9 L43 | L47 A12 L48 L51 A15 L52 A14 L53 A13 L54 L49 A11 L50 A10 | L55 A45 L56 A46 L57 A44 L58 A43 | L59 A42 L60 A41 L61 A40 L62 A39 | L66 A48 L92 A70 L105 L108 A73 L107 A72 L106 A71 L109 L93 A47 | L67 A57 L94 A59 L95 A60 L96 A58 | L68 L74 A50 L75 A51 L73 L76 A88 L127 A89 L72 L69 A49 L70 A69 L104 A67 | L77 A85 L123 L125 A86 L126 A87 L124 A84 L80 L78 A53 L79 A52 | L81 A54 L82 L84 L87 L83 A77 L110 A76 | L82 L83 L87 L84 | L85 L90 L91 L86 A68 L87 L83 | L90 A55 L89 A56 L88 L85 | L85 L86 L91 L90 | A63 L100 A64 L99 A62 L98 A61 L97 | L101 A66 L102 A65 L103 L116 A83 L117 L119 A81 L120 A80 L121 L118 L115 A82 | L111 A74 L112 A79 L114 A78 L113 A75 | L128 A90 L129 A93 L131 A92 L130 A91 | L132 A95 L158 A117 L171 L174 A120 L173 A119 L172 A118 L175 L159 A94 | L134 L140 A97 L141 A98 L139 L142 A135 L193 A136 L138 L135 A96 L136 A116 L170 A114 | L143 A132 L189 L191 A133 L192 A134 L190 A131 L146 L144 A100 L145 A99 | L147 A101 L148 L150 L153 L149 A124 L176 A123 | L148 L149 L153 L150 | L151 L156 L157 L152 A115 L153 L149 | L156 A102 L155 A103 L154 L151 | L151 L152 L157 L156 | A110 L166 A111 L165 A109 L164 A108 L163 | L167 A113 L168 A112 L169 L182 A130 L183 L185 A128 L186 A127 L187 L184 L181 A129 | L177 A121 L178 A126 L180 A125 L179 A122 | L198 A142 L224 A164 L237 L240 A167 L239 A166 L238 A165 L241 L225 A141 | L199 A151 L226 A153 L227 A154 L228 A152 | L213 A148 L214 L216 L219 L215 A171 L242 A170 | L214 L215 L219 L216 | L217 L222 L223 L218 A162 L219 L215 | L222 A149 L221 A150 L220 L217 | L217 L218 L223 L222 | L243 A168 L244 A173 L246 A172 L245 A169 | L260 A184 L261 A187 L263 A186 L262 A185
